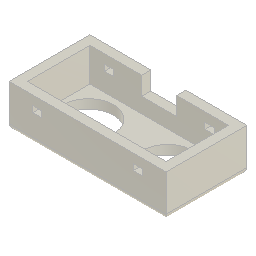
HC-SR04 Cradle (Autodesk Fusion 360 design; units mm, degrees)
Autodesk Fusion 360 part; units mm, degrees
sketch "Sketch1" plane through (0, 0, 0) normal (0, 0, 1) x (1, 0, 0)
  line L0 (0, 0) -> (51.5, 0)
  line L1 (51.5, 0) -> (51.5, 26.5)
  line L2 (51.5, 26.5) -> (0, 26.5)
  line L3 (0, 26.5) -> (0, 0)
  line L4 (3, 3) -> (48.5, 3)
  line L5 (48.5, 3) -> (48.5, 23.5)
  line L6 (48.5, 23.5) -> (3, 23.5)
  line L7 (3, 23.5) -> (3, 3)
  circle A0 centre (12.75, 13.25) radius 8.25
  circle A1 centre (38.75, 13.25) radius 8.25
  dimension "d1" = 51.5
  dimension "d2" = 26.5
  dimension "d3" = -3
  dimension "d4" = 16.5
  dimension "d5" = 16.5
  dimension "d6" = 26
  dimension "d7" = 13.25
  dimension "d8" = 12.75
  constraint horizontal L0
  constraint vertical L1
  constraint horizontal L2
  constraint vertical L3
  constraint coincident L0.start L3.end
  measures "d1" distance of L0.start L0.end
  measures "d2" distance of L0.start L2.end
  measures "d4" diameter of A0
  measures "d5" diameter of A1
  measures "d6" distance of A0.centre A1.centre
  measures "d7" distance of L0 A0.centre
  measures "d8" distance of L3 A0.centre
extrude "Extrude1" add sketch "Sketch1" along normal blind 3 contours L4 L5 L6 L7
extrude "Extrude2" add sketch "Sketch1" along normal blind 14 contours L0 L1 L2 L3
sketch "Sketch2" plane through (0, 0, 14) normal (0, 0, 1) x (-1, 0, 0)
  line L0 (-3, -3) -> (-3, -23.5)
  line L1 (-3, -23.5) -> (-48.5, -23.5)
  line L2 (-48.5, -23.5) -> (-48.5, -3)
  line L3 (-48.5, -3) -> (-3, -3)
  line L4 (0, -26.5) -> (0, 0)
  line L5 (0, 0) -> (-51.5, 0)
  line L6 (-51.5, 0) -> (-51.5, -26.5)
  line L7 (-51.5, -26.5) -> (0, -26.5)
  line L8 (-20, -26.5) -> (-31.5, -26.5)
  line L9 (-31.5, -26.5) -> (-31.5, -23.5)
  line L10 (-31.5, -23.5) -> (-20, -23.5)
  line L11 (-20, -23.5) -> (-20, -26.5)
  dimension "d13" = 20
  dimension "d14" = 20
  constraint horizontal L8
  constraint vertical L9
  constraint horizontal L10
  constraint vertical L11
  constraint coincident L1 L9.end
  constraint coincident L7 L8.start
  measures "d13" distance of L4 L11
  measures "d14" distance of L6 L9
extrude "Extrude3" cut sketch "Sketch2" against normal blind 6 contours L1 L7 L8 L9 L10 L11
sketch "Sketch3" plane through (0, 0, 0) normal (0, -1, 0) x (1, 0, 0)
  line L0 (0, 0) -> (51.5, 0)
  line L1 (51.5, 0) -> (51.5, 14)
  line L2 (51.5, 14) -> (0, 14)
  line L3 (0, 14) -> (0, 0)
  line L4 (7.75, 11) -> (10.75, 11)
  line L5 (10.75, 11) -> (10.75, 9)
  line L6 (10.75, 9) -> (7.75, 9)
  line L7 (7.75, 9) -> (7.75, 11)
  line L8 (40.75, 11) -> (43.75, 11)
  line L9 (43.75, 11) -> (43.75, 9)
  line L10 (43.75, 9) -> (40.75, 9)
  line L11 (40.75, 9) -> (40.75, 11)
  dimension "d18" = 3
  dimension "d19" = 2
  dimension "d20" = 30
  dimension "d21" = 51.5
  dimension "d22" = 10.75
  dimension "d23" = 3
  constraint horizontal L4
  constraint vertical L5
  constraint horizontal L6
  constraint vertical L7
  constraint horizontal L8
  constraint vertical L9
  constraint horizontal L10
  constraint vertical L11
  constraint collinear L4 L8
  constraint collinear L6 L10
  constraint equal L4 L8
  measures "d18" distance of L5.end L6.end
  measures "d19" distance of L4.start L6.end
  measures "d20" distance of L5 L11
  measures "d21" distance of L0.start L0.end
  measures "d22" distance of L3 L5
  measures "d23" distance of L2 L4
extrude "Extrude4" cut sketch "Sketch3" against normal up to surface (26.5 mm away) contours L4 L5 L6 L7 | L8 L9 L10 L11
fillet "Fillet1" radius 2 4 edges at (25.75, 0, 0) (0, 13.25, 0) (25.75, 26.5, 0) (51.5, 13.25, 0)
equation "d1 = 45 mm + 3 mm + 3 mm + 0.5 mm"
equation "d2 = 20 mm + 3 mm + 3 mm + 0.5 mm"
equation "d4 = 16 mm + 0.5 mm"
equation "d5 = 16 mm + 0.5 mm"
equation "d7 = d2 / 2"
equation "d8 = ( d1 - d6 ) / 2"
equation "d11 = 10 mm + 3 mm + 1 mm"
equation "d14 = d13"
equation "d22 = ( d21 - d20 ) / 2"
